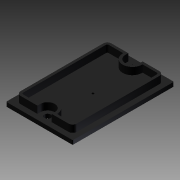
# Autodesk Inventor part: Goma
Saved by Autodesk Inventor 2016 (Build 200138000, 138)
## iProperties
Created: 2013-07-10
Part Number: Goma
Material: Generic
Document SubType Name: Modeling
Designer: Luis
Density: 1 g/cm^3
Appearance: Glossy - Black
Author: Luis
Autodesk Inventor part; units mm, degrees
ref_plane "YZ Plane" through (0, 0, 0) normal (1, 0, 0) x (0, 1, 0)
ref_plane "XZ Plane" through (0, 0, 0) normal (0, 1, 0) x (-1, 0, 0)
ref_plane "XY Plane" through (0, 0, 0) normal (0, 0, 1) x (1, 0, 0)
sketch "Sketch1" plane through (0, 0, 0) normal (0, 0, 1) x (1, 0, 0)
  circle A0 centre (-1.4563, -20.8) radius 1.5
  circle A1 centre (-1.4563, 20.8) radius 1.5
  line L0 (14.8852, 24.5) -> (14.8852, -24.5)
  arc A2 (14.8852, 24.5) -> (14.5437, 24.8416) centre (14.5437, 24.5) ccw
  line L1 (-17.4563, 24.8416) -> (14.5437, 24.8416)
  arc A3 (-17.4563, 24.8416) -> (-17.7979, 24.5) centre (-17.4563, 24.5) ccw
  line L2 (-17.7979, -24.5) -> (-17.7979, 24.5)
  arc A4 (-17.7979, -24.5) -> (-17.4563, -24.8416) centre (-17.4563, -24.5) ccw
  line L3 (14.5437, -24.8416) -> (-17.4563, -24.8416)
  arc A5 (14.5437, -24.8416) -> (14.8852, -24.5) centre (14.5437, -24.5) ccw
  line L4 (-13.2563, 22.3) -> (-4.9563, 22.3)
  line L5 (-4.9563, 22.3) -> (-4.9563, 20.8)
  arc A6 (-4.9563, 20.8) -> (2.0437, 20.8) centre (-1.4563, 20.8) ccw
  line L6 (2.0437, 20.8) -> (2.0437, 22.3)
  line L7 (2.0437, 22.3) -> (10.3437, 22.3)
  arc A7 (12.3437, 20.3) -> (10.3437, 22.3) centre (10.3437, 20.3) ccw
  line L8 (12.3437, 20.3) -> (12.3437, -20.3)
  arc A8 (10.3437, -22.3) -> (12.3437, -20.3) centre (10.3437, -20.3) ccw
  line L9 (10.3437, -22.3) -> (2.0437, -22.3)
  line L10 (2.0437, -22.3) -> (2.0437, -20.8)
  arc A9 (2.0437, -20.8) -> (-4.9563, -20.8) centre (-1.4563, -20.8) ccw
  line L11 (-4.9563, -20.8) -> (-4.9563, -22.3)
  line L12 (-4.9563, -22.3) -> (-13.2563, -22.3)
  arc A10 (-15.2563, -20.3) -> (-13.2563, -22.3) centre (-13.2563, -20.3) ccw
  line L13 (-15.2563, -20.3) -> (-15.2563, 20.3)
  arc A11 (-13.2563, 22.3) -> (-15.2563, 20.3) centre (-13.2563, 20.3) ccw
  circle A12 centre (-1.4563, 20.8) radius 1.5
  circle A13 centre (-1.4563, -20.8) radius 1.5
  arc A14 (-17.4563, 26.5) -> (-19.4563, 24.5) centre (-17.4563, 24.5) ccw
  line L14 (-19.4563, -24.5) -> (-19.4563, 24.5)
  arc A15 (-19.4563, -24.5) -> (-17.4563, -26.5) centre (-17.4563, -24.5) ccw
  line L15 (14.5437, -26.5) -> (-17.4563, -26.5)
  arc A16 (14.5437, -26.5) -> (16.5437, -24.5) centre (14.5437, -24.5) ccw
  line L16 (16.5437, 24.5) -> (16.5437, -24.5)
  arc A17 (16.5437, 24.5) -> (14.5437, 26.5) centre (14.5437, 24.5) ccw
  line L17 (-17.4563, 26.5) -> (14.5437, 26.5)
  arc A18 (-6.2217, 20.8) -> (3.3091, 20.8) centre (-1.4563, 20.8) ccw
  line L18 (-6.2217, 20.8) -> (-6.2217, 21.0346)
  line L19 (-6.2217, 21.0346) -> (-13.2563, 21.0346)
  arc A19 (-13.2563, 21.0346) -> (-13.9909, 20.3) centre (-13.2563, 20.3) ccw
  line L20 (-13.9909, 20.3) -> (-13.9909, -20.3)
  arc A20 (-13.9909, -20.3) -> (-13.2563, -21.0346) centre (-13.2563, -20.3) ccw
  line L21 (-13.2563, -21.0346) -> (-6.2217, -21.0346)
  line L22 (-6.2217, -21.0346) -> (-6.2217, -20.8)
  arc A21 (3.3091, -20.8) -> (-6.2217, -20.8) centre (-1.4563, -20.8) ccw
  line L23 (3.3091, -20.8) -> (3.3091, -21.0346)
  line L24 (3.3091, -21.0346) -> (10.3437, -21.0346)
  arc A22 (10.3437, -21.0346) -> (11.0783, -20.3) centre (10.3437, -20.3) ccw
  line L25 (11.0783, -20.3) -> (11.0783, 20.3)
  arc A23 (11.0783, 20.3) -> (10.3437, 21.0346) centre (10.3437, 20.3) ccw
  line L26 (10.3437, 21.0346) -> (3.3091, 21.0346)
  line L27 (3.3091, 21.0346) -> (3.3091, 20.8)
  point P0 (0, 0)
  point P1 (0, 0)
  point P2 (0, 0)
  constraints: 56 end point, 40 point on circle, 24 centre point, 15 other
extrude "Extrusion1" add sketch "Sketch1" along normal blind 2 contours L0 A5 L3 A4 L2 A3 L1 A2
extrude "Extrusion2" add sketch "Sketch1" along normal blind 5.5 contours L4 L5 A6 L6 L7 A7 L8 A8 L9 L10 A9 L11 L12 A10 L13 A11
extrude "Extrusion3" add sketch "Sketch1" along normal blind 2 contours A18 L27 L26 A23 L25 A22 L24 L23 A21 L22 L21 A20 L20 A19 L19 L18
sketch "Sketch2" plane through (0, 0, 2) normal (0, 0, 1) x (1, 0, 0)
  circle A0 centre (0, 0) radius 0.5
  dimension "d6" = 1
  constraints: 1 centre point, 1 coincident
  measures "d6" diameter of A0
extrude "Extrusion4" cut sketch "Sketch2" along normal through all both and the other way through all
body "Solid1"
